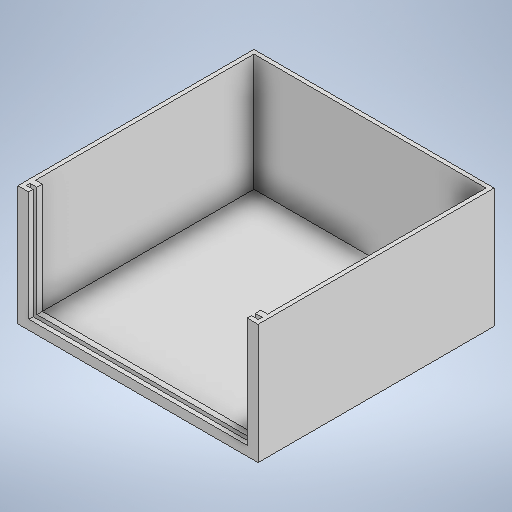
# Autodesk Inventor part: Box
Saved by Autodesk Inventor 2025 (Build 290162000, 162)
## iProperties
Created: 2024-08-10
Part Number: Box
Material: Generic
Document SubType Name: Modeling
Designer: ethan
Density: 1 g/cm^3
Appearance: Default
Author: ethan
Autodesk Inventor part; units mm, degrees
ref_plane "YZ Plane" through (0, 0, 0) normal (1, 0, 0) x (0, 1, 0)
ref_plane "XZ Plane" through (0, 0, 0) normal (0, 1, 0) x (-1, 0, 0)
ref_plane "XY Plane" through (0, 0, 0) normal (0, 0, 1) x (1, 0, 0)
sketch "Sketch1" plane through (0, 0, 0) normal (0, 0, 1) x (1, 0, 0)
  line L0 (0, 0) -> (170.5, 0)
  line L1 (170.5, 0) -> (170.5, 86)
  line L2 (170.5, 86) -> (0, 86)
  line L3 (0, 86) -> (0, 0)
  line L4 (5, 5) -> (165.5, 5)
  line L5 (165.5, 5) -> (165.5, 81)
  line L6 (165.5, 81) -> (5, 81)
  line L7 (5, 81) -> (5, 5)
  line L8 (5, 81) -> (5, 86)
  line L9 (165.5, 81) -> (165.5, 86)
  dimension "d0" = 170.5
  dimension "d1" = 86
  dimension "d2" = 5
  constraints: 20 end point, 4 parallel, 3 perpendicular, 3 point on line, 1 horizontal, 3 other
  measures "d0" distance of L2.end L1.end
  measures "d1" distance of L1.end L0.end
  measures "d2" distance between parallel lines of L3 L7
extrude "Extrusion1" add sketch "Sketch1" along normal blind 4 contours L3 L2 L8 L7 L4 L5 L9 L1 L0
sketch "Sketch2" plane through (0, 0, 0) normal (0, -1, 0) x (1, 0, 0)
  line L0 (0, 0) -> (170.5, 0) construction
  line L1 (170.5, 0) -> (0, 0) construction
  line L2 (0, 0) -> (0, -6) construction
  line L3 (0, -6) -> (170.5, -6) construction
  line L4 (170.5, -6) -> (170.5, 0) construction
  line L5 (170.5, -6) -> (0, -6) construction
  line L6 (0, -6) -> (0, 164.5) construction
  line L7 (0, 164.5) -> (170.5, 164.5) construction
  line L8 (170.5, 164.5) -> (170.5, -6) construction
  line L9 (170.5, -6) -> (0, -6)
  line L10 (0, -6) -> (0, 164.5)
  line L11 (0, 164.5) -> (170.5, 164.5)
  line L12 (170.5, 164.5) -> (170.5, -6)
  dimension "d5" = 6
  dimension "d6" = 170.5
  dimension "d7" = 170.5
  constraints: 24 end point, 6 parallel, 3 horizontal, 3 perpendicular
  measures "d5" distance of L2.end L1.end
  measures "d6" distance of L6.end L7.end
  measures "d7" distance of L5.end L6.end
extrude "Extrusion2" add sketch "Sketch2" along normal blind 2
sketch "Sketch3" plane through (170.5, 0, -6) normal (0, 0, -1) x (-1, 0, 0)
  line L0 (0, 86) -> (5, 86) projected
  line L1 (0, 0) -> (0, 86) projected
  line L2 (170.5, 0) -> (0, 0) projected
  line L3 (170.5, 86) -> (170.5, 0) projected
  line L4 (165.5, 86) -> (170.5, 86) projected
  line L5 (165.5, 5) -> (165.5, 86) projected
  line L6 (5, 5) -> (165.5, 5) projected
  line L7 (5, 86) -> (5, 5) projected
extrude "Extrusion3" add sketch "Sketch3" against normal blind 3.2
sketch "Sketch4" plane through (0, 0, 0) normal (-1, 0, 0) x (0, 0, 1)
  line L0 (0, 86) -> (0, 0) construction
  line L1 (4, 86) -> (4, 0) construction
  line L2 (0, 86) -> (4, 86) construction
  line L3 (-6, 86) -> (164.5, 86)
  line L4 (164.5, 86) -> (164.5, -2)
  line L5 (164.5, -2) -> (-6, -2)
  line L6 (-6, -2) -> (-6, 86)
  line L7 (0, 0) -> (-2.8, 0) projected
  line L8 (-2.8, 86) -> (-2.8, 0) projected
  line L9 (-6, 86) -> (-2.8, 86) projected
  line L10 (-6, 86) -> (-6, -2) projected
  line L11 (164.5, -2) -> (-6, -2) projected
  line L12 (164.5, 0) -> (164.5, -2) projected
  line L13 (164.5, 0) -> (4, 0) projected
  constraints: 8 end point, 2 parallel, 1 horizontal, 1 perpendicular
extrude "Extrusion4" add sketch "Sketch4" along normal blind 3
sketch "Sketch5" plane through (170.5, 0, 0) normal (1, 0, 0) x (0, 0, -1)
  line L0 (6, -2) -> (-164.5, -2) projected
  line L1 (-164.5, 86) -> (-4, 86) projected
  line L2 (6, -2) -> (-164.5, -2)
  line L3 (-164.5, -2) -> (-164.5, 86)
  line L4 (-164.5, 86) -> (6, 86)
  line L5 (6, 86) -> (6, -2)
  point P0 (0, 0)
  point P1 (-4, 86)
  constraints: 8 end point, 2 parallel, 1 horizontal, 1 perpendicular
extrude "Extrusion5" add sketch "Sketch5" along normal blind 3
sketch "Sketch6" plane through (0, 0, 164.5) normal (0, 0, 1) x (1, 0, 0)
  line L0 (-3, -2) -> (-3, 86) projected
  line L1 (173.5, 86) -> (173.5, -2) projected
  line L2 (-3, -2) -> (173.5, -2)
  line L3 (173.5, -2) -> (173.5, 86)
  line L4 (173.5, 86) -> (-3, 86)
  line L5 (-3, 86) -> (-3, -2)
  point P0 (0, 0)
  point P1 (173.5, -2)
  point P2 (-3, 86)
  constraints: 8 end point, 2 parallel, 1 horizontal, 1 perpendicular
extrude "Extrusion6" add sketch "Sketch6" along normal blind 3
body "Solid1"
